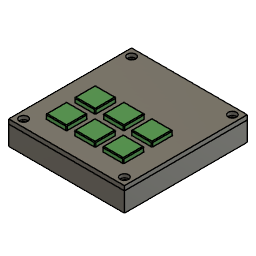
PCB SOURCE FILES (Autodesk Fusion 360 design; units mm, degrees)
part number: 2026-01-23-20-00-59-580
Autodesk Fusion 360 part; units mm, degrees
sketch "pcb visual" plane through (0, 0, 0) normal (0, 1, 0) x (1, 0, 0)
  line L0 (0, 0) -> (57.5, 0)
  line L1 (57.5, 0) -> (57.5, 62.29)
  line L2 (57.5, 62.29) -> (0, 62.29)
  line L3 (0, 62.29) -> (0, 0)
  dimension "d1" = 57.5
  dimension "d2" = 62.29
  constraint horizontal L0
  constraint vertical L1
  constraint horizontal L2
  constraint vertical L3
  constraint coincident L0.start L3.end
  measures "d1" distance of L0.start L0.end
  measures "d2" distance of L0.start L2.end
extrude "Extrude1" add sketch "pcb visual" along normal blind 1.6 makes body 1
sketch "base" plane through (0, 0, 0) normal (0, 1, 0) x (1, 0, 0)
  line L0 (0, 0) -> (-10, 0)
  line L1 (-10, 0) -> (-10, -10)
  line L2 (-10, -10) -> (67.5, -10)
  line L3 (67.5, -10) -> (67.5, 72.29)
  line L4 (67.5, 72.29) -> (-10, 72.29)
  line L5 (-10, 72.29) -> (-10, -10)
  line L6 (0, 0) -> (57.5, 0)
  line L7 (57.5, 0) -> (57.5, 62.29)
  line L8 (57.5, 62.29) -> (0, 62.29)
  line L9 (0, 62.29) -> (0, 0)
  line L10 (-10, 72.29) -> (-5, 72.29)
  line L11 (67.5, 72.29) -> (62.5, 72.29)
  line L12 (62.5, 72.29) -> (62.5, 67.29)
  circle A0 centre (62.5, 67.29) radius 1.45
  line L13 (67.5, -10) -> (62.5, -10)
  line L14 (62.5, -10) -> (62.5, -5)
  circle A1 centre (62.5, -5) radius 1.45
  line L15 (-10, -10) -> (-10, -5)
  line L16 (-10, -5) -> (-5, -5)
  circle A2 centre (-5, -5) radius 1.45
  line L17 (-5, 72.29) -> (-5, 67.29)
  circle A3 centre (-5, 67.29) radius 1.45
  dimension "d5" = 10
  dimension "d6" = 10
  dimension "d7" = 77.5
  dimension "d8" = 82.29
  dimension "d9" = 57.5
  dimension "d10" = 62.29
  dimension "d11" = 5
  dimension "d14" = 5
  dimension "d15" = 5
  dimension "d16" = 2.9
  dimension "d17" = 5
  dimension "d18" = 5
  dimension "d19" = 2.9
  dimension "d20" = 5
  dimension "d21" = 5
  dimension "d22" = 2.9
  dimension "d42" = 5
  dimension "d43" = 2.9
  constraint coincident L0.start L6.start
  constraint horizontal L0
  constraint perpendicular L0 L1
  constraint horizontal L2
  constraint vertical L3
  constraint horizontal L4
  constraint vertical L5
  constraint horizontal L6
  constraint vertical L7
  constraint horizontal L8
  constraint vertical L9
  constraint perpendicular L5 L10
  constraint perpendicular L3 L11
  constraint perpendicular L4 L12
  constraint coincident L12.end A0.centre
  constraint perpendicular L3 L13
  constraint perpendicular L2 L14
  constraint coincident L14.end A1.centre
  constraint perpendicular L2 L15
  constraint perpendicular L1 L16
  constraint coincident L16.end A2.centre
  constraint perpendicular L10 L17
  constraint coincident L17.end A3.centre
  measures "d5" distance of L0.start L0.end
  measures "d6" distance of L0.end L1.end
  measures "d7" distance of L1.end L2.end
  measures "d8" distance of L1.end L4.end
  measures "d9" distance of L0.start L6.end
  measures "d10" distance of L0.start L8.end
  measures "d11" distance of L4.end L10.end
  measures "d14" distance of L3.end L11.end
  measures "d15" distance of L11.end L12.end
  measures "d16" diameter of A0
  measures "d17" distance of L2.end L13.end
  measures "d18" distance of L13.end L14.end
  measures "d19" diameter of A1
  measures "d20" distance of L1.end L15.end
  measures "d21" distance of L15.end L16.end
  measures "d22" diameter of A2
  measures "d42" distance of L10.end L17.end
  measures "d43" diameter of A3
move_body "Move1" bodies 1 to x (1, 0, 0) y (0, 1, 0) z (0, 0, 1) at (0, 40, 0)
move_body "Move2" bodies 1 to x (1, 0, 0) y (0, 1, 0) z (0, 0, 1) at (0, -37, 0)
extrude "Extrude5" add sketch "base" along normal blind 3 separate body contours L6 L7 L8 L9 makes body 2
extrude "Extrude6" add sketch "base" along normal blind 13 bodies 2
sketch "cover" plane through (0, 0, 0) normal (0, 1, 0) x (1, 0, 0)
  line L0 (0, 0) -> (0, -10)
  line L1 (0, -10) -> (-10, -10)
  line L2 (-10, -10) -> (72.29, -10)
  line L3 (72.29, -10) -> (72.29, 67.5)
  line L4 (72.29, 67.5) -> (-10, 67.5)
  line L5 (-10, 67.5) -> (-10, -10)
  line L6 (-10, -10) -> (-10, -5)
  line L7 (-10, 67.5) -> (-10, 62.5)
  line L8 (72.29, 67.5) -> (72.29, 62.5)
  line L9 (72.29, -10) -> (72.29, -5)
  line L10 (-10, -10) -> (-10, -5)
  line L11 (-10, -10) -> (-10, -5)
  line L12 (-10, -5) -> (-5, -5)
  line L13 (72.29, -10) -> (72.29, -5)
  line L14 (72.29, -5) -> (67.29, -5)
  circle A0 centre (67.29, -5) radius 1.45
  circle A1 centre (-5, -5) radius 1.45
  line L15 (72.29, 67.5) -> (67.29, 67.5)
  line L16 (67.29, 67.5) -> (67.29, 62.5)
  circle A2 centre (67.29, 62.5) radius 1.45
  line L17 (-10, 67.5) -> (-10, 62.5)
  line L18 (-10, 62.5) -> (-5, 62.5)
  circle A3 centre (-5, 62.5) radius 1.45
  dimension "d71" = 10
  dimension "d72" = 82.29
  dimension "d73" = 77.5
  dimension "d88" = 5
  dimension "d89" = 5
  dimension "d90" = 5
  dimension "d91" = 5
  dimension "d92" = 2.9
  dimension "d93" = 2.9
  dimension "d94" = 5
  dimension "d95" = 5
  dimension "d96" = 2.9
  dimension "d97" = 5
  dimension "d98" = 5
  dimension "d99" = 2.9
  constraint coincident L0.start origin
  constraint vertical L0
  constraint perpendicular L0 L1
  constraint horizontal L2
  constraint vertical L3
  constraint horizontal L4
  constraint vertical L5
  constraint perpendicular L1 L6
  constraint perpendicular L4 L7
  constraint perpendicular L4 L8
  constraint perpendicular L2 L9
  constraint perpendicular L2 L11
  constraint perpendicular L10 L12
  constraint perpendicular L2 L13
  constraint perpendicular L13 L14
  constraint coincident L14.end A0.centre
  constraint coincident L12.end A1.centre
  constraint perpendicular L8 L15
  constraint perpendicular L4 L16
  constraint coincident L16.end A2.centre
  constraint perpendicular L4 L17
  constraint perpendicular L17 L18
  constraint coincident L18.end A3.centre
  measures "d71" distance of L0.end L1.end
  measures "d72" distance of L1.end L2.end
  measures "d73" distance of L1.end L4.end
  measures "d88" distance of L1.end L6.end
  measures "d89" distance of L6.end L12.end
  measures "d90" distance of L2.end L9.end
  measures "d91" distance of L9.end L14.end
  measures "d92" diameter of A0
  measures "d93" diameter of A1
  measures "d94" distance of L3.end L15.end
  measures "d95" distance of L15.end L16.end
  measures "d96" diameter of A2
  measures "d97" distance of L4.end L7.end
  measures "d98" distance of L7.end L18.end
  measures "d99" diameter of A3
move_body "Move3" bodies 2 to x (1, 0, 0) y (0, 1, 0) z (0, 0, 1) at (0, 100, 0)
move_body "Move4" bodies 1 to x (1, 0, 0) y (0, 1, 0) z (0, 0, 1) at (0, 100, 0)
move_body "Move6" bodies 1 to x (1, 0, 0) y (0, 1, 0) z (0, 0, 1) at (0, -100, 0)
move_body "Move7" bodies 2 to x (1, 0, 0) y (0, 1, 0) z (0, 0, 1) at (0, -100, 0)
move_body "Move8" bodies 1 to x (1, 0, 0) y (0, 1, 0) z (0, 0, 1) at (0, 100, 0)
move_body "Move9" bodies 2 to x (1, 0, 0) y (0, 1, 0) z (0, 0, 1) at (0, 100, 0)
extrude "Extrude11" add sketch "cover" along normal blind 3 separate body makes body 3
move_body "Move10" bodies 3 to x (1, 0, 0) y (0, 1, 0) z (0, 0, 1) at (0, 10, 0)
move_body "Move11" bodies 1 to x (1, 0, 0) y (0, 1, 0) z (0, 0, 1) at (0, -100, 0)
move_body "Move12" bodies 2 to x (1, 0, 0) y (0, 1, 0) z (0, 0, 1) at (0, -100, 0)
move_body "Move13" bodies 3 to x (0, 0, -1) y (0, 1, 0) z (1, 0, 0) at (57.5, 0, -77.5)
move_body "Move14" bodies 3 to x (1, 0, 0) y (0, 1, 0) z (0, 0, 1) at (0, 0, 77.5)
move_body "Move15" bodies 3 to x (1, 0, 0) y (0, 1, 0) z (0, 0, 1) at (0, 3, 0)
sketch "keycapholes" plane through (0, 0, 0) normal (0, 1, 0) x (-1, 0, 0)
  circle A0 centre (-62.5, 5) radius 1.45
  circle A1 centre (5, -67.29) radius 1.45
  circle A2 centre (-62.5, -67.29) radius 1.45
  circle A3 centre (5, 5) radius 1.45
  line L0 (10, -72.29) -> (10, 10)
  line L1 (10, 10) -> (-67.5, 10)
  line L2 (-67.5, 10) -> (-67.5, -72.29)
  line L3 (-67.5, -72.29) -> (10, -72.29)
  line L4 (10, 10) -> (0, 10)
  line L5 (0, 10) -> (0, 0)
  line L6 (0, 0) -> (-57.5, 0)
  line L7 (-57.5, 0) -> (-57.5, -62.29)
  line L8 (-57.5, -62.29) -> (0, -62.29)
  line L9 (0, -62.29) -> (0, 0)
  line L10 (0, 0) -> (-2.54, 0)
  line L11 (0, 0) -> (-2.54, 0)
  line L12 (0, 0) -> (0, -2.54)
  line L13 (0, -2.54) -> (-2.54, -2.54) construction
  line L14 (-2.54, -2.54) -> (-2.8936, -2.8936) construction
  line L15 (-2.8936, -2.8936) -> (-2.3936, -2.8936) construction
  line L16 (-2.8936, -2.8936) -> (-2.8936, -2.3936) construction
  arc A4 (-2.3936, -2.8936) -> (-2.8936, -2.3936) centre (-2.8936, -2.8936) ccw
  line L17 (-2.3936, -2.8936) -> (-2.3936, -15.8936)
  line L18 (-2.8936, -2.3936) -> (-15.8936, -2.3936)
  line L19 (-2.3936, -15.8936) -> (-2.8936, -15.8936) construction
  line L20 (-2.8936, -15.8936) -> (-2.8936, -16.3936) construction
  arc A5 (-2.8936, -16.3936) -> (-2.3936, -15.8936) centre (-2.8936, -15.8936) ccw
  line L21 (-2.8936, -16.3936) -> (-15.8936, -16.3936)
  line L22 (-15.8936, -16.3936) -> (-15.8936, -15.8936) construction
  line L23 (-15.8936, -15.8936) -> (-16.3936, -15.8936) construction
  arc A6 (-16.3936, -15.8936) -> (-15.8936, -16.3936) centre (-15.8936, -15.8936) ccw
  line L24 (-16.3936, -15.8936) -> (-16.3936, -2.8936)
  line L25 (-15.8936, -2.3936) -> (-15.8936, -2.8936) construction
  line L26 (-15.8936, -2.8936) -> (-16.3936, -2.8936) construction
  arc A7 (-15.8936, -2.3936) -> (-16.3936, -2.8936) centre (-15.8936, -2.8936) ccw
  line L27 (-15.8936, -16.3936) -> (-16.3936, -16.3936) construction
  line L28 (-16.3936, -16.3936) -> (-18.9286, -16.3936) construction
  line L29 (-18.9286, -16.3936) -> (-18.9286, -15.3936) construction
  line L30 (-21.4636, -15.8936) -> (-21.4636, -2.8936)
  arc A8 (-21.9636, -16.3936) -> (-21.4636, -15.8936) centre (-21.9636, -15.8936) ccw
  line L31 (-34.9636, -16.3936) -> (-21.9636, -16.3936)
  arc A9 (-35.4636, -15.8936) -> (-34.9636, -16.3936) centre (-34.9636, -15.8936) ccw
  line L32 (-35.4636, -2.8936) -> (-35.4636, -15.8936)
  arc A10 (-34.9636, -2.3936) -> (-35.4636, -2.8936) centre (-34.9636, -2.8936) ccw
  line L33 (-34.9636, -2.3936) -> (-21.9636, -2.3936)
  arc A11 (-21.4636, -2.8936) -> (-21.9636, -2.3936) centre (-21.9636, -2.8936) ccw
  line L34 (-34.9636, -15.8936) -> (-34.9636, -16.3936) construction
  line L35 (-34.9636, -16.3936) -> (-35.4636, -16.3936) construction
  line L36 (-35.4636, -16.3936) -> (-37.9836, -16.3936) construction
  line L37 (-37.9836, -16.3936) -> (-37.9836, -15.3936) construction
  line L38 (-40.5036, -2.8936) -> (-40.5036, -15.8936)
  arc A12 (-41.0036, -16.3936) -> (-40.5036, -15.8936) centre (-41.0036, -15.8936) ccw
  line L39 (-41.0036, -16.3936) -> (-54.0036, -16.3936)
  arc A13 (-54.5036, -15.8936) -> (-54.0036, -16.3936) centre (-54.0036, -15.8936) ccw
  line L40 (-54.5036, -15.8936) -> (-54.5036, -2.8936)
  arc A14 (-54.0036, -2.3936) -> (-54.5036, -2.8936) centre (-54.0036, -2.8936) ccw
  line L41 (-41.0036, -2.3936) -> (-54.0036, -2.3936)
  arc A15 (-40.5036, -2.8936) -> (-41.0036, -2.3936) centre (-41.0036, -2.8936) ccw
  line L42 (-16.3936, -16.3936) -> (-16.3936, -18.9936) construction
  line L43 (-16.3936, -18.9936) -> (-16.15, -18.9936) construction
  line L44 (-2.8936, -21.5936) -> (-15.8936, -21.5936)
  line L45 (-2.3936, -35.0936) -> (-2.3936, -22.0936)
  arc A16 (-2.3936, -22.0936) -> (-2.8936, -21.5936) centre (-2.8936, -22.0936) ccw
  arc A17 (-15.8936, -21.5936) -> (-16.3936, -22.0936) centre (-15.8936, -22.0936) ccw
  line L46 (-16.3936, -22.0936) -> (-16.3936, -35.0936)
  arc A18 (-16.3936, -35.0936) -> (-15.8936, -35.5936) centre (-15.8936, -35.0936) ccw
  line L47 (-2.8936, -35.5936) -> (-15.8936, -35.5936)
  arc A19 (-2.8936, -35.5936) -> (-2.3936, -35.0936) centre (-2.8936, -35.0936) ccw
  line L48 (-15.8936, -35.0936) -> (-15.8936, -35.5936) construction
  line L49 (-15.8936, -35.5936) -> (-16.3936, -35.5936) construction
  line L50 (-16.3936, -35.5936) -> (-18.9736, -35.5936) construction
  line L51 (-18.9736, -35.5936) -> (-18.9736, -34.7) construction
  line L52 (-21.5536, -22.0936) -> (-21.5536, -35.0936)
  arc A20 (-22.0536, -35.5936) -> (-21.5536, -35.0936) centre (-22.0536, -35.0936) ccw
  line L53 (-35.0536, -35.5936) -> (-22.0536, -35.5936)
  arc A21 (-35.5536, -35.0936) -> (-35.0536, -35.5936) centre (-35.0536, -35.0936) ccw
  line L54 (-35.5536, -35.0936) -> (-35.5536, -22.0936)
  arc A22 (-35.0536, -21.5936) -> (-35.5536, -22.0936) centre (-35.0536, -22.0936) ccw
  line L55 (-35.0536, -21.5936) -> (-22.0536, -21.5936)
  arc A23 (-21.5536, -22.0936) -> (-22.0536, -21.5936) centre (-22.0536, -22.0936) ccw
  line L56 (-54.0036, -15.8936) -> (-54.0036, -16.3936) construction
  line L57 (-54.0036, -16.3936) -> (-54.5036, -16.3936) construction
  line L58 (-54.5036, -16.3936) -> (-54.5036, -18.9936) construction
  line L59 (-54.5036, -18.9936) -> (-51.7, -18.9936) construction
  line L60 (-41.0036, -21.5936) -> (-54.0036, -21.5936)
  arc A24 (-40.5036, -22.0936) -> (-41.0036, -21.5936) centre (-41.0036, -22.0936) ccw
  line L61 (-40.5036, -35.0936) -> (-40.5036, -22.0936)
  arc A25 (-41.0036, -35.5936) -> (-40.5036, -35.0936) centre (-41.0036, -35.0936) ccw
  line L62 (-41.0036, -35.5936) -> (-54.0036, -35.5936)
  arc A26 (-54.5036, -35.0936) -> (-54.0036, -35.5936) centre (-54.0036, -35.0936) ccw
  line L63 (-54.5036, -22.0936) -> (-54.5036, -35.0936)
  arc A27 (-54.0036, -21.5936) -> (-54.5036, -22.0936) centre (-54.0036, -22.0936) ccw
  dimension "d102" = 10
  dimension "d103" = 10
  dimension "d104" = 57.5
  dimension "d105" = 62.29
  dimension "d129" = 2.54
  dimension "d130" = 2.54
  dimension "d131" = 0.5
  dimension "d132" = 0.5
  dimension "d133" = 0.5
  dimension "d134" = 13
  dimension "d135" = 13
  dimension "d136" = 0.5
  dimension "d137" = 0.5
  dimension "d138" = 13
  dimension "d139" = 0.5
  dimension "d140" = 0.5
  dimension "d141" = 13
  dimension "d142" = 0.5
  dimension "d143" = 2.535
  dimension "d144" = 1
  dimension "d145" = 0.5
  dimension "d146" = 2.52
  dimension "d147" = 1
  dimension "d148" = 2.6
  dimension "d149" = 0.5
  dimension "d150" = 2.58
  dimension "d151" = 0.5
  dimension "d152" = 2.6
  constraint coincident L0.end L1.start
  constraint perpendicular L0 L4
  constraint perpendicular L1 L5
  constraint horizontal L6
  constraint vertical L7
  constraint horizontal L8
  constraint vertical L9
  constraint coincident L5.end L6.start
  constraint perpendicular L5 L10
  constraint perpendicular L10 L12
  constraint perpendicular L12 L13
  constraint horizontal L15
  constraint perpendicular L15 L16
  constraint tangent A4 L17
  constraint perpendicular L15 L17
  constraint perpendicular L16 L18
  constraint perpendicular L17 L19
  constraint perpendicular L19 L20
  constraint perpendicular L20 L21
  constraint perpendicular L21 L22
  constraint perpendicular L22 L23
  constraint perpendicular L23 L24
  constraint perpendicular L18 L25
  constraint perpendicular L24 L26
  constraint perpendicular L22 L27
  constraint parallel L27 L28
  constraint perpendicular L28 L29
  constraint symmetric L15.end L29 L32.start
  constraint symmetric L16.end L29 A10.start
  constraint symmetric A4 L29 A10
  constraint symmetric L17.end L29 A9.start
  constraint symmetric L18.end L29 L33.end
  constraint symmetric L20.end L29 L31.start
  constraint symmetric A5 L29 A9
  constraint symmetric L21.end L29 A8.start
  constraint symmetric L23.end L29 L30.start
  constraint symmetric A6 L29 A8
  constraint symmetric L24.end L29 L30.end
  constraint symmetric A7 L29 A11
  constraint coincident A9.centre L34.start
  constraint perpendicular L31 L34
  constraint perpendicular L34 L35
  constraint parallel L35 L36
  constraint perpendicular L36 L37
  constraint symmetric L30.start L37 A13.start
  constraint symmetric L30.end L37 L40.end
  constraint symmetric A8.start L37 L39.end
  constraint symmetric A8 L37 A13
  constraint symmetric L31.start L37 A12.start
  constraint symmetric A9.start L37 L38.end
  constraint symmetric A9 L37 A12
  constraint symmetric L32.start L37 L38.start
  constraint symmetric A10.start L37 L41.start
  constraint symmetric A10 L37 A15
  constraint symmetric L33.end L37 A14.start
  constraint symmetric A11 L37 A14
  constraint perpendicular L27 L42
  constraint perpendicular L42 L43
  constraint symmetric L15.end L43 L45.start
  constraint symmetric L16.end L43 L47.start
  constraint symmetric A4 L43 A19
  constraint symmetric L17.end L43 L45.end
  constraint symmetric L18.end L43 A18.end
  constraint symmetric L20.end L43 L44.start
  constraint symmetric A5 L43 A16
  constraint symmetric L21.end L43 L44.end
  constraint symmetric L23.end L43 A17.end
  constraint symmetric A6 L43 A17
  constraint symmetric L24.end L43 L46.end
  constraint symmetric A7 L43 A18
  constraint coincident A18.centre L48.start
  constraint perpendicular L47 L48
  constraint perpendicular L48 L49
  constraint horizontal L50
  constraint perpendicular L50 L51
  constraint symmetric L44.start L51 A22.start
  constraint symmetric L44.end L51 L55.end
  constraint symmetric L45.start L51 A21.start
  constraint symmetric L45.end L51 L54.end
  constraint symmetric A16 L51 A22
  constraint symmetric A17.end L51 L52.start
  constraint symmetric A17 L51 A23
  constraint symmetric L46.end L51 L52.end
  constraint symmetric A18.end L51 A20.start
  constraint symmetric A18 L51 A20
  constraint symmetric L47.start L51 L53.start
  constraint symmetric A19 L51 A21
  constraint coincident A13.centre L56.start
  constraint perpendicular L39 L56
  constraint perpendicular L56 L57
  constraint perpendicular L57 L58
  constraint perpendicular L58 L59
  constraint symmetric L38.start L59 L61.start
  constraint symmetric L38.end L59 A24.start
  constraint symmetric A12.start L59 L60.start
  constraint symmetric A12 L59 A24
  constraint symmetric L39.end L59 L60.end
  constraint symmetric A13.start L59 L63.start
  constraint symmetric A13 L59 A27
  constraint symmetric L40.end L59 A26.start
  constraint symmetric A14.start L59 L62.end
  constraint symmetric A14 L59 A26
  constraint symmetric L41.start L59 A25.start
  constraint symmetric A15 L59 A25
  measures "d102" distance of L0.end L4.end
  measures "d103" distance of L4.end L5.end
  measures "d104" distance of L5.end L6.end
  measures "d105" distance of L5.end L8.end
  measures "d129" distance of L5.end L12.end
  measures "d130" distance of L12.end L13.end
  measures "d131" distance of L13.end L14.end
  measures "d132" distance of L14.end L15.end
  measures "d133" distance of L14.end L16.end
  measures "d134" distance of L15.end L17.end
  measures "d135" distance of L16.end L18.end
  measures "d136" distance of L17.end L19.end
  measures "d137" distance of L19.end L20.end
  measures "d138" distance of L20.end L21.end
  measures "d139" distance of L21.end L22.end
  measures "d140" distance of L22.end L23.end
  measures "d141" distance of L23.end L24.end
  measures "d142" distance of L21.end L27.end
  measures "d143" distance of L27.end L28.end
  measures "d144" distance of L28.end L29.end
  measures "d145" distance of L31.start L35.end
  measures "d146" distance of L35.end L36.end
  measures "d147" distance of L36.end L37.end
  measures "d148" distance of L27.end L42.end
  measures "d149" distance of A18.end L49.end
  measures "d150" distance of L49.end L50.end
  measures "d151" distance of L39.end L57.end
  measures "d152" distance of L57.end L58.end
move_body "Move16" bodies 1 to x (1, 0, 0) y (0, 1, 0) z (0, 0, 1) at (0, 100, 0)
move_body "Move17" bodies 2 to x (1, 0, 0) y (0, 1, 0) z (0, 0, 1) at (0, 100, 0)
move_body "Move18" bodies 3 to x (1, 0, 0) y (0, 1, 0) z (0, 0, 1) at (0, -10, 0)
move_body "Move19" bodies 3 to x (1, 0, 0) y (0, 1, 0) z (0, 0, 1) at (0, -3, 0)
extrude "Extrude13" cut sketch "keycapholes" along normal blind 3 contours A4 L17 L18 A5 L21 A6 L24 A7 | L30 A8 L31 A9 L32 A10 L33 A11 | L38 A12 L39 A13 L40 A14 L41 A15 | L44 L45 A16 A17 L46 A18 L47 A19 | L52 A20 L53 A21 L54 A22 L55 A23 | L60 A24 L61 A25 L62 A26 L63 A27 bodies 3
move_body "Move20" bodies 3 to x (1, 0, 0) y (0, 1, 0) z (0, 0, 1) at (0, 13, 0)
move_body "Move21" bodies 1 to x (1, 0, 0) y (0, 1, 0) z (0, 0, 1) at (0, -100, 0)
move_body "Move22" bodies 2 to x (1, 0, 0) y (0, 1, 0) z (0, 0, 1) at (0, -100, 0)
sketch "microcontroller" plane through (0, 0, -72.29) normal (0, 0, -1) x (-1, 0, 0)
  line L0 (-67.5, 0) -> (10, 0)
  line L1 (10, 0) -> (10, 13)
  line L2 (10, 13) -> (-67.5, 13)
  line L3 (-67.5, 13) -> (-67.5, 0)
  line L4 (-67.5, 13) -> (-28.75, 13)
  line L5 (-28.75, 13) -> (-37.65, 13)
  line L6 (-28.75, 13) -> (-19.85, 13)
  line L7 (-37.65, 13) -> (-37.65, 4.6)
  line L8 (-37.65, 4.6) -> (-19.85, 4.6)
  line L9 (-19.85, 4.6) -> (-19.85, 13)
  line L10 (-19.85, 13) -> (-37.65, 13)
  line L11 (-37.65, 13) -> (-37.65, 4.6)
  dimension "d157" = 38.75
  dimension "d158" = 8.9
  dimension "d159" = 8.9
  dimension "d160" = 8.4
  constraint coincident L2.end L3.start
  constraint perpendicular L3 L4
  constraint parallel L4 L5
  constraint parallel L2 L6
  constraint perpendicular L5 L7
  constraint horizontal L8
  constraint vertical L9
  constraint horizontal L10
  constraint vertical L11
  measures "d157" distance of L2.end L4.end
  measures "d158" distance of L4.end L5.end
  measures "d159" distance of L4.end L6.end
  measures "d160" distance of L5.end L7.end
extrude "Extrude14" cut sketch "microcontroller" against normal blind 10 contours L2 L4 L5 L6 L7 L8 L9 L10 L11 bodies 2
sketch "countersink" plane through (0, 16, 0) normal (0, 1, 0) x (-1, 0, 0)
  line L0 (-34.9636, -2.3936) -> (-21.9636, -2.3936)
  arc A0 (-21.4636, -2.8936) -> (-21.9636, -2.3936) centre (-21.9636, -2.8936) ccw
  line L1 (-21.4636, -2.8936) -> (-21.4636, -15.8936)
  arc A1 (-21.9636, -16.3936) -> (-21.4636, -15.8936) centre (-21.9636, -15.8936) ccw
  line L2 (-21.9636, -16.3936) -> (-34.9636, -16.3936)
  arc A2 (-35.4636, -15.8936) -> (-34.9636, -16.3936) centre (-34.9636, -15.8936) ccw
  line L3 (-35.4636, -15.8936) -> (-35.4636, -2.8936)
  arc A3 (-34.9636, -2.3936) -> (-35.4636, -2.8936) centre (-34.9636, -2.8936) ccw
  line L4 (-2.3936, -2.8936) -> (-2.3936, -15.8936)
  arc A4 (-2.8936, -16.3936) -> (-2.3936, -15.8936) centre (-2.8936, -15.8936) ccw
  line L5 (-2.8936, -16.3936) -> (-15.8936, -16.3936)
  arc A5 (-16.3936, -15.8936) -> (-15.8936, -16.3936) centre (-15.8936, -15.8936) ccw
  line L6 (-16.3936, -15.8936) -> (-16.3936, -2.8936)
  arc A6 (-15.8936, -2.3936) -> (-16.3936, -2.8936) centre (-15.8936, -2.8936) ccw
  line L7 (-15.8936, -2.3936) -> (-2.8936, -2.3936)
  arc A7 (-2.3936, -2.8936) -> (-2.8936, -2.3936) centre (-2.8936, -2.8936) ccw
  line L8 (-41.0036, -16.3936) -> (-54.0036, -16.3936)
  arc A8 (-54.5036, -15.8936) -> (-54.0036, -16.3936) centre (-54.0036, -15.8936) ccw
  line L9 (-54.5036, -15.8936) -> (-54.5036, -2.8936)
  arc A9 (-54.0036, -2.3936) -> (-54.5036, -2.8936) centre (-54.0036, -2.8936) ccw
  line L10 (-54.0036, -2.3936) -> (-41.0036, -2.3936)
  arc A10 (-40.5036, -2.8936) -> (-41.0036, -2.3936) centre (-41.0036, -2.8936) ccw
  line L11 (-40.5036, -2.8936) -> (-40.5036, -15.8936)
  arc A11 (-41.0036, -16.3936) -> (-40.5036, -15.8936) centre (-41.0036, -15.8936) ccw
  line L12 (-35.5536, -35.0936) -> (-35.5536, -22.0936)
  arc A12 (-35.0536, -21.5936) -> (-35.5536, -22.0936) centre (-35.0536, -22.0936) ccw
  line L13 (-35.0536, -21.5936) -> (-22.0536, -21.5936)
  arc A13 (-21.5536, -22.0936) -> (-22.0536, -21.5936) centre (-22.0536, -22.0936) ccw
  line L14 (-21.5536, -22.0936) -> (-21.5536, -35.0936)
  arc A14 (-22.0536, -35.5936) -> (-21.5536, -35.0936) centre (-22.0536, -35.0936) ccw
  line L15 (-22.0536, -35.5936) -> (-35.0536, -35.5936)
  arc A15 (-35.5536, -35.0936) -> (-35.0536, -35.5936) centre (-35.0536, -35.0936) ccw
  line L16 (-2.8936, -35.5936) -> (-15.8936, -35.5936)
  arc A16 (-16.3936, -35.0936) -> (-15.8936, -35.5936) centre (-15.8936, -35.0936) ccw
  line L17 (-16.3936, -35.0936) -> (-16.3936, -22.0936)
  arc A17 (-15.8936, -21.5936) -> (-16.3936, -22.0936) centre (-15.8936, -22.0936) ccw
  line L18 (-15.8936, -21.5936) -> (-2.8936, -21.5936)
  arc A18 (-2.3936, -22.0936) -> (-2.8936, -21.5936) centre (-2.8936, -22.0936) ccw
  line L19 (-2.3936, -22.0936) -> (-2.3936, -35.0936)
  arc A19 (-2.8936, -35.5936) -> (-2.3936, -35.0936) centre (-2.8936, -35.0936) ccw
  line L20 (-41.0036, -35.5936) -> (-54.0036, -35.5936)
  arc A20 (-54.5036, -35.0936) -> (-54.0036, -35.5936) centre (-54.0036, -35.0936) ccw
  line L21 (-54.5036, -35.0936) -> (-54.5036, -22.0936)
  arc A21 (-54.0036, -21.5936) -> (-54.5036, -22.0936) centre (-54.0036, -22.0936) ccw
  line L22 (-54.0036, -21.5936) -> (-41.0036, -21.5936)
  arc A22 (-40.5036, -22.0936) -> (-41.0036, -21.5936) centre (-41.0036, -22.0936) ccw
  line L23 (-40.5036, -22.0936) -> (-40.5036, -35.0936)
  arc A23 (-41.0036, -35.5936) -> (-40.5036, -35.0936) centre (-41.0036, -35.0936) ccw
  circle A24 centre (-62.5, 5) radius 1.45
  circle A25 centre (5, -67.29) radius 1.45
  circle A26 centre (-62.5, -67.29) radius 1.45
  circle A27 centre (5, 5) radius 1.45
  line L24 (10, -72.29) -> (10, 10)
  line L25 (10, 10) -> (-67.5, 10)
  line L26 (-67.5, 10) -> (-67.5, -72.29)
  line L27 (-67.5, -72.29) -> (10, -72.29)
  line L28 (10, 10) -> (-67.5, 10)
  line L29 (-67.5, 10) -> (-67.5, -72.29)
  line L30 (-67.5, -72.29) -> (10, -72.29)
  line L31 (10, -72.29) -> (10, 10)
  line L32 (10, 10) -> (5, 10)
  line L33 (5, 10) -> (5, 5)
  circle A28 centre (5, 5) radius 2.775
  line L34 (-67.5, 10) -> (-62.5, 10)
  line L35 (-62.5, 10) -> (-62.5, 5)
  circle A29 centre (-62.5, 5) radius 2.775
  line L36 (-67.5, -72.29) -> (-62.5, -72.29)
  line L37 (-62.5, -72.29) -> (-62.5, -67.29)
  circle A30 centre (-62.5, -67.29) radius 2.775
  line L38 (10, -72.29) -> (5, -72.29)
  line L39 (5, -72.29) -> (5, -67.29)
  circle A31 centre (5, -67.29) radius 2.775
  dimension "d163" = 5
  dimension "d164" = 5
  dimension "d165" = 5.55
  dimension "d166" = 5
  dimension "d167" = 5.55
  dimension "d168" = 5
  dimension "d169" = 5.55
  dimension "d170" = 5
  dimension "d171" = 5
  dimension "d172" = 5.55
  constraint horizontal L28
  constraint vertical L29
  constraint horizontal L30
  constraint vertical L31
  constraint coincident L26.end L27.start
  constraint coincident L24.end L25.start
  constraint perpendicular L31 L32
  constraint perpendicular L28 L33
  constraint concentric A27 A28
  constraint coincident L25.end L26.start
  constraint perpendicular L26 L34
  constraint coincident A24.centre L35.end
  constraint perpendicular L29 L36
  constraint coincident A26.centre L37.end
  constraint concentric A26 A30
  constraint coincident L24.start L27.end
  constraint perpendicular L24 L38
  constraint perpendicular L30 L39
  constraint concentric A25 A31
  measures "d163" distance of L24.end L32.end
  measures "d164" distance of L32.end A27.centre
  measures "d165" diameter of A28
  measures "d166" distance of L25.end L34.end
  measures "d167" diameter of A29
  measures "d168" distance of L26.end L36.end
  measures "d169" diameter of A30
  measures "d170" distance of L24.start L38.end
  measures "d171" distance of L38.end A25.centre
  measures "d172" diameter of A31
extrude "Extrude15" cut sketch "countersink" against normal blind 2.4 contours A28 | A29 | A30 | A31 bodies 3
sketch "Sketch13" plane through (0, 0, 0) normal (0, 1, 0) x (1, 0, 0)
  line L0 (-0.1626, 0) -> (13.8374, 0)
  line L1 (13.8374, 0) -> (13.8374, 14)
  line L2 (13.8374, 14) -> (-0.1626, 14)
  line L3 (-0.1626, 14) -> (-0.1626, 0)
  line L4 (-0.1626, 0) -> (0.3374, 0) construction
  line L5 (0.3374, 0) -> (0.3374, 0.5) construction
  line L6 (0.3374, 0.5) -> (-0.1626, 0.5) construction
  line L7 (-0.1626, 0.5) -> (-0.1626, 0) construction
  arc A0 (-0.1626, 0.5) -> (0.3374, 0) centre (0.3374, 0.5) ccw
  line L8 (13.8374, 0) -> (13.3374, 0) construction
  line L9 (13.3374, 0) -> (13.3374, 0.5) construction
  line L10 (13.3374, 0.5) -> (13.8374, 0.5) construction
  line L11 (13.8374, 0.5) -> (13.8374, 0) construction
  arc A1 (13.3374, 0) -> (13.8374, 0.5) centre (13.3374, 0.5) ccw
  line L12 (13.8374, 14) -> (13.3374, 14) construction
  line L13 (13.3374, 14) -> (13.3374, 13.5) construction
  line L14 (13.3374, 13.5) -> (13.8374, 13.5) construction
  line L15 (13.8374, 13.5) -> (13.8374, 14)
  arc A2 (13.8374, 13.5) -> (13.3374, 14) centre (13.3374, 13.5) ccw
  line L16 (-0.1626, 14) -> (0.3374, 14) construction
  line L17 (0.3374, 14) -> (0.3374, 13.5) construction
  line L18 (0.3374, 13.5) -> (-0.1626, 13.5) construction
  line L19 (-0.1626, 13.5) -> (-0.1626, 14) construction
  arc A3 (0.3374, 14) -> (-0.1626, 13.5) centre (0.3374, 13.5) ccw
  dimension "d175" = 14
  dimension "d176" = 14
  dimension "d177" = 0.5
  dimension "d178" = 0.5
  dimension "d179" = 0.5
  dimension "d180" = 0.5
  dimension "d181" = 0.5
  dimension "d182" = 0.5
  dimension "d183" = 0.5
  dimension "d184" = 0.5
  constraint horizontal L0
  constraint vertical L1
  constraint horizontal L2
  constraint vertical L3
  constraint horizontal L4
  constraint vertical L5
  constraint horizontal L6
  constraint vertical L7
  constraint coincident L5.end L6.start
  constraint horizontal L8
  constraint vertical L9
  constraint horizontal L10
  constraint vertical L11
  constraint horizontal L12
  constraint vertical L13
  constraint horizontal L14
  constraint vertical L15
  constraint horizontal L16
  constraint vertical L17
  constraint horizontal L18
  constraint vertical L19
  measures "d175" distance of L0.start L0.end
  measures "d176" distance of L0.start L2.end
  measures "d177" distance of L0.start L4.end
  measures "d178" distance of L0.start L6.end
  measures "d179" distance of L0.end L8.end
  measures "d180" distance of L0.end L10.end
  measures "d181" distance of L1.end L12.end
  measures "d182" distance of L1.end L14.end
  measures "d183" distance of L2.end L16.end
  measures "d184" distance of L2.end L18.end
extrude "Extrude16" add sketch "Sketch13" along normal blind 6 separate body contours L0 L1 L2 L3 A0 A1 A2 A3 makes body 4
fillet "Fillet1" radius 0.5 8 faces at (13.3612, 2, -0.0006) (13.8374, 4, -9.1667) (13.7704, 4, -13.75) (9.0041, 2, -14) (-0.0956, 4, -13.75) (-0.1626, 4, -4.8333) (0.3136, 4, -0.0006) (4.6707, 2, 0) on bodies 4
move_body "Move23" bodies 4 to x (1, 0, 0) y (0, 1, 0) z (0, 0, 1) at (0, 16, 0)
move_body "Move24" bodies 4 to x (1, 0, 0) y (0, 1, 0) z (0, 0, 1) at (2.556, 0, 0)
move_body "Move25" bodies 4 to x (1, 0, 0) y (0, 1, 0) z (0, 0, 1) at (0, -3, 0)
move_body "Move26" bodies 4 to x (1, 0, 0) y (0, 1, 0) z (0, 0, 1) at (0, 0, -2.394)
copy_body "CopyPasteBodies1" bodies 4 makes body 5
move_body "Move27" bodies 5 to x (1, 0, 0) y (0, 1, 0) z (0, 0, 1) at (0, 0, -19.1502)
move_body "Move28" bodies 5 to x (1, 0, 0) y (0, 1, 0) z (0, 0, 1) at (0, 0, -0.0373)
copy_body "CopyPasteBodies2" bodies 4 makes body 6
move_body "Move29" bodies 6 to x (1, 0, 0) y (0, 1, 0) z (0, 0, 1) at (19.2383, 0, 0)
move_body "Move30" bodies 6 to x (1, 0, 0) y (0, 1, 0) z (0, 0, 1) at (-0.1687, 0, 0)
copy_body "CopyPasteBodies3" bodies 6 makes body 7
move_body "Move31" bodies 7 to x (1, 0, 0) y (0, 1, 0) z (0, 0, 1) at (18.8598, 0, 0)
copy_body "CopyPasteBodies4" bodies 7 makes body 8
move_body "Move32" bodies 8 to x (1, 0, 0) y (0, 1, 0) z (0, 0, 1) at (0.1249, 0, -18.3308)
move_body "Move33" bodies 8 to x (1, 0, 0) y (0, 1, 0) z (0, 0, 1) at (0, 0, -0.7383)
copy_body "CopyPasteBodies5" bodies 6 makes body 9
move_body "Move34" bodies 9 to x (1, 0, 0) y (0, 1, 0) z (0, 0, 1) at (0.0891, 0, -18.3522)
move_body "Move35" bodies 9 to x (1, 0, 0) y (0, 1, 0) z (0, 0, 1) at (0, 0, -0.8692)
move_body "Move36" bodies 2 to x (1, 0, 0) y (0, 1, 0) z (0, 0, 1) at (-80, 0, 0)
move_body "Move37" bodies 1 to x (1, 0, 0) y (0, 1, 0) z (0, 0, 1) at (-80, 0, 0)
move_body "Move38" bodies 2 to x (1, 0, 0) y (0, 1, 0) z (0, 0, 1) at (80, 0, 0)
move_body "Move39" bodies 1 to x (1, 0, 0) y (0, 1, 0) z (0, 0, 1) at (80, 0, 0)
named bodies: "pcb", "base", "top", "key top right", "key bottom right", "key top middle", "key top left", "key bottom left", "key bottom middle"
